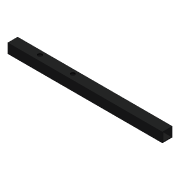
# Autodesk Inventor part: KétvégenMartSzelvény
Saved by Autodesk Inventor 2015 SP1 (Build 190203100, 203)
## iProperties
Created: 2014-08-08
Part Number: KétvégenMartSzelvény
Material: Acetal Resin, Black
Document SubType Name: Modeling
Designer: laca
Density: 1.425 g/cm^3
Appearance: Smooth - Black
Mass: 54.2497 g
Surface Area: 509.22 cm^2
Volume: 38.07 cm^3
Author: laca
Autodesk Inventor part; units mm, degrees
ref_plane "YZ Plane" through (0, 0, 0) normal (1, 0, 0) x (0, 1, 0)
ref_plane "XZ Plane" through (0, 0, 0) normal (0, 1, 0) x (-1, 0, 0)
ref_plane "XY Plane" through (0, 0, 0) normal (0, 0, 1) x (1, 0, 0)
sketch "Sketch1" plane through (0, 0, 0) normal (1, 0, 0) x (0, 1, 0)
  line L0 (0, 0) -> (12, 0)
  line L1 (12, 0) -> (12, 12)
  line L2 (12, 12) -> (0, 12)
  line L3 (0, 12) -> (0, 0)
  line L4 (-1.5, 13.5) -> (13.5, 13.5)
  line L5 (13.5, 13.5) -> (13.5, -1.5)
  line L6 (13.5, -1.5) -> (-1.5, -1.5)
  line L7 (-1.5, -1.5) -> (-1.5, 13.5)
  dimension "d0" = 1.5
  dimension "d1" = 12
  dimension "d2" = 12
  constraints: 16 end point, 4 parallel, 2 perpendicular, 1 horizontal, 3 other
  measures "d0" distance between parallel lines of L4 L2
  measures "d1" distance of L2.end L0.start
  measures "d2" distance of L0.start L0.end
extrude "Extrusion1" add sketch "Sketch1" along normal blind 235
sketch "Sketch11" plane through (0, 13.5, 13.5) normal (0, 1, 0) x (1, 0, 0)
  point P0 (90.9, 8)
  point P1 (40.9, 8)
hole "Hole11" at (90.9, 13.5, 5.5) at (40.9, 13.5, 5.5) direction (0, -1, 0) diameter 6.6 depth 1.5
sketch "Sketch12" plane through (0, -1.5, -1.5) normal (0, -1, 0) x (1, 0, 0)
  point P0 (90.9, 7)
  point P1 (40.9, 7)
hole "Hole13" at (90.9, -1.5, 5.5) at (40.9, -1.5, 5.5) direction (0, 1, 0) diameter 6.6 depth 1.5
equation "\"d0\" = ZártSzelvényFalVastagság"
equation "\"d1\" = ZártSzelvényBelsőÁtmérő"
equation "\"d2\" = ZártSzelvényBelsőÁtmérő"
equation "\"ZártSzelvényFalVastagság\" = 1.5"
equation "\"ZártSzelvényBelsőÁtmérő\" = 12"
equation "\"CsapágyHázKülsőÁtmérő\" = 32"
equation "\"ZártSzelvényKülsőÁtmérő\" = 15"
equation "\"CsapágyBelsőÁtmérő\" = 12"
equation "\"CsapágyKülsőÁtmérő\" = 28"
equation "\"CsapágyHázBelsőÁtmérő\" = 26"
equation "\"CsapágyHázHoszza\" = 45"
equation "\"CsapágySzélesége\" = 8"
body "Solid1"
